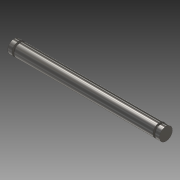
# Autodesk Inventor part: phalanx_1_mcp_tendon_shaft
Saved by Autodesk Inventor 2017 SP1 (Build 210196100, 196)
## iProperties
Created: 2017-06-26
Part Number: phalanx_1_mcp_tendon_shaft
Material: Generic
Document SubType Name: Modeling
Designer: Tomasz
Density: 1 g/cm^3
Appearance: Steel - Polished
Author: Tomasz
Autodesk Inventor part; units mm, degrees
ref_plane "YZ Plane" through (0, 0, 0) normal (1, 0, 0) x (0, 1, 0)
ref_plane "XZ Plane" through (0, 0, 0) normal (0, 1, 0) x (-1, 0, 0)
ref_plane "XY Plane" through (0, 0, 0) normal (0, 0, 1) x (1, 0, 0)
sketch "Sketch1" plane through (0, 0, 0) normal (0, 0, 1) x (1, 0, 0)
  line L0 (-21.6, 1) -> (0, 1)
  line L1 (0, 0) -> (0, 10.9873) construction
  line L2 (-21.9, 1) -> (-21.9, 1)
  line L3 (-21.9, 1) -> (-22.6, 1)
  line L4 (-22.6, 1) -> (-22.6, 0)
  line L5 (-22.6, 0) -> (1, 0)
  line L6 (0, 1) -> (0, 0.7)
  line L7 (0, 0.7) -> (0.3, 0.7)
  line L8 (0.3, 0.7) -> (0.3, 1)
  line L9 (0.3, 1) -> (1, 1)
  line L10 (1, 1) -> (1, 0)
  line L11 (1, 0) -> (0, 0)
  line L12 (-21.6, 1) -> (-21.6, 0.7)
  line L13 (-21.6, 0.7) -> (-21.9, 0.7)
  line L14 (-21.9, 0.7) -> (-21.9, 1)
  dimension "d7" = 0.3
  dimension "d8" = 0.3
  dimension "d9" = 1
  dimension "d12" = 2
  dimension "d13" = 21.6
  dimension "d14" = 0.3
  dimension "d15" = 1
  constraints: 30 end point, 10 perpendicular, 4 point on line, 2 collinear, 2 vertical, 1 horizontal
  measures "d7" distance between parallel lines of L7 L0
  measures "d8" distance between parallel lines of L8 L1
  measures "d9" distance between parallel lines of L1 L10
  measures "d12" diameter of L0 L5
  measures "d13" distance between parallel lines of L6 L12
  measures "d14" distance between parallel lines of L12 L14
  measures "d15" distance between parallel lines of L12 L4
revolve "Revolution1" add sketch "Sketch1" angle 360 about axis through (-22.6, 0, 0) along (1, 0, 0)
equation "\"d14\" = d7"
equation "\"d15\" = d9"
equation "\"finger_inner_width\" = 14"
body "Solid1"
